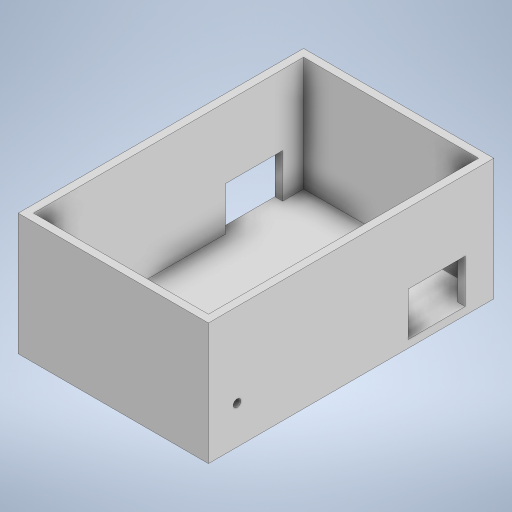
# Autodesk Inventor part: эвакуатор
Saved by Autodesk Inventor 2023.2 (Build 272271000, 271)
## iProperties
Created: 2024-01-18
Part Number: эвакуатор
Material: Типовые
Document SubType Name: Modeling
Designer: парпа
Density: 1 g/cm^3
Appearance: По умолчанию
Author: парпа
Autodesk Inventor part; units mm, degrees
ref_plane "YZ Plane" through (0, 0, 0) normal (1, 0, 0) x (0, 1, 0)
ref_plane "XZ Plane" through (0, 0, 0) normal (0, 1, 0) x (-1, 0, 0)
ref_plane "XY Plane" through (0, 0, 0) normal (0, 0, 1) x (1, 0, 0)
sketch "Эскиз1" plane through (0, 0, 0) normal (0, 1, 0) x (-1, 0, 0)
  line L0 (-50, 75) -> (50, 75)
  line L1 (50, 75) -> (50, -75)
  line L2 (50, -75) -> (-50, -75)
  line L3 (-50, -75) -> (-50, 75)
  line L4 (-50, 75) -> (50, -75) construction
  line L5 (50, 75) -> (-50, -75) construction
  point P0 (0, 0)
  dimension "d0" = 150
  dimension "d1" = 100
  constraints: 12 end point, 2 midpoint, 2 parallel, 1 horizontal, 1 perpendicular
  measures "d0" distance of L0.end L1.end
  measures "d1" distance of L1.end L2.end
extrude "Выдавливание1" add sketch "Эскиз1" along normal blind 4
sketch "Эскиз2" plane through (0, 4, 0) normal (0, 1, 0) x (1, 0, 0)
  line L0 (50, 75) -> (-50, 75) projected
  line L1 (50, -75) -> (-50, -75)
  line L2 (-50, -75) -> (-50, 75)
  line L3 (-50, 75) -> (50, 75)
  line L4 (50, 75) -> (50, -75)
  line L5 (50, -75) -> (-50, 75) construction
  line L6 (-50, -75) -> (50, 75) construction
  line L7 (46, -71) -> (-46, -71)
  line L8 (-46, -71) -> (-46, 71)
  line L9 (-46, 71) -> (46, 71)
  line L10 (46, 71) -> (46, -71)
  line L11 (46, -71) -> (-46, 71) construction
  line L12 (-46, -71) -> (46, 71) construction
  point P0 (0, 0)
  dimension "d4" = 4
  dimension "d5" = 4
  constraints: 24 end point, 4 midpoint, 4 parallel, 2 horizontal, 2 perpendicular
  measures "d4" distance between parallel lines of L2 L8
  measures "d5" distance between parallel lines of L7 L1
extrude "Выдавливание2" add sketch "Эскиз2" along normal blind 60
sketch "Эскиз3" plane through (50, 0, 75) normal (1, 0, 0) x (0, 0, -1)
  line L0 (150, 0) -> (0, 0) projected
  circle A0 centre (15, 20) radius 2
  point P0 (75, 0)
  dimension "d10" = 4
  constraints: 1 centre point
  measures "d10" diameter of A0
extrude "Выдавливание3" cut sketch "Эскиз3" against normal blind 135.5
sketch "Эскиз4" plane through (50, 0, 75) normal (1, 0, 0) x (0, 0, -1)
  line L0 (150, 0) -> (0, 0) projected
  line L1 (146, 4) -> (4, 4) projected
  line L2 (135, 4) -> (105, 4)
  line L3 (105, 4) -> (105, 27)
  line L4 (105, 27) -> (135, 27)
  line L5 (135, 27) -> (135, 4)
  point P0 (75, 0)
  dimension "d14" = 23
  dimension "d15" = 30
  constraints: 8 end point, 2 parallel, 1 horizontal, 1 perpendicular, 1 point on line
  measures "d14" distance of L4.end L2.start
  measures "d15" distance of L3.end L4.end
extrude "Выдавливание4" cut sketch "Эскиз4" against normal blind 135.5
